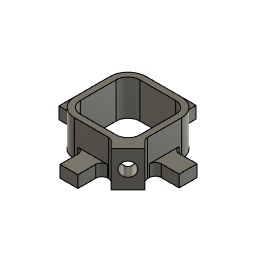
Miniscope_v4_Baseplate_Var_2 (Autodesk Fusion 360 design; units mm, degrees)
Autodesk Fusion 360 part; units mm, degrees
sketch "Sketch1" plane through (0, 0, 0) normal (0, 1, 0) x (1, 0, 0)
  line L0 (1.5, -2) -> (-1.5, -2)
  line L1 (-2, -1.5) -> (-2, 1.5)
  line L2 (-1.5, 2) -> (1.5, 2)
  line L3 (2, 1.5) -> (2, -1.5)
  line L4 (2, -2) -> (-2, 2) construction
  line L5 (-2, -2) -> (2, 2) construction
  line L6 (-1.5, -3) -> (1.5858, -3)
  line L7 (3, -1.5858) -> (3, 1.5)
  line L8 (1.5, 3) -> (-1.5, 3)
  line L9 (-3, 1.5) -> (-3, -1.5)
  line L10 (-3, -3) -> (3, 3) construction
  line L11 (3, -3) -> (-2.9939, 2.9939) construction
  arc A0 (-1.5, 2) -> (-2, 1.5) centre (-1.5, 1.5) ccw
  arc A1 (-2, -1.5) -> (-1.5, -2) centre (-1.5, -1.5) ccw
  arc A2 (1.5, -2) -> (2, -1.5) centre (1.5, -1.5) ccw
  arc A3 (2, 1.5) -> (1.5, 2) centre (1.5, 1.5) ccw
  arc A4 (-1.5, 3) -> (-3, 1.5) centre (-1.5, 1.5) ccw
  arc A5 (-3, -1.5) -> (-1.5, -3) centre (-1.5, -1.5) ccw
  arc A6 (3, 1.5) -> (1.5, 3) centre (1.5, 1.5) ccw
  line L12 (3.7071, -2.2929) -> (2.2929, -3.7071)
  line L13 (2.2929, -3.7071) -> (1.5858, -3)
  line L14 (3, -1.5858) -> (3.7071, -2.2929)
  dimension "d1" = 4
  dimension "d2" = 4
  dimension "d3" = 0.5
  dimension "d4" = 6
  dimension "d5" = 6
  dimension "d6" = 1.5
  dimension "d7" = 2
  dimension "d31" = 2
  dimension "d32" = 3
  constraint perpendicular L0 L1
  constraint parallel L0 L2
  constraint parallel L1 L3
  constraint horizontal L0
  constraint coincident L4 origin
  constraint coincident L5 origin
  constraint perpendicular L6 L7
  constraint parallel L6 L8
  constraint parallel L7 L9
  constraint horizontal L6
  constraint coincident L10 origin
  constraint coincident L11 origin
  constraint coincident L4.end L2
  constraint coincident L4.end L1
  constraint tangent L2 A0
  constraint tangent L1 A0
  constraint coincident L5.start L1
  constraint coincident L5.start L0
  constraint tangent L1 A1
  constraint tangent L0 A1
  constraint equal A0 A1
  constraint tangent L0 A2
  constraint tangent L3 A2
  constraint equal A0 A2
  constraint coincident L5.end L3
  constraint coincident L5.end L2
  constraint tangent L3 A3
  constraint tangent L2 A3
  constraint equal A0 A3
  constraint tangent L8 A4
  constraint tangent L9 A4
  constraint coincident L10.start L9
  constraint coincident L10.start L6
  constraint tangent L9 A5
  constraint tangent L6 A5
  constraint equal A4 A5
  constraint coincident L11.start L6
  constraint coincident L11.start L7
  constraint coincident L10.end L7
  constraint coincident L10.end L8
  constraint tangent L7 A6
  constraint tangent L8 A6
  constraint equal A4 A6
  constraint perpendicular L12 L13
  constraint parallel L13 L14
  constraint midpoint L11.start L12
  constraint parallel L11 L13
  constraint coincident L7.start L14.start
  constraint coincident L6.end L13.end
  measures "d1" distance of L5.start L4.end
  measures "d2" distance of L4.end L5.end
  measures "d3" radius of A0
  measures "d4" distance of L10.start L11.start
  measures "d5" distance of L11.start L10.end
  measures "d6" radius of A4
  measures "d7" distance of L12.start L12.end
  measures "d31" distance of L1 origin
  measures "d32" distance of origin L8
extrude "Extrude1" add sketch "Sketch1" along normal blind 2.5
sketch "Sketch2" plane through (3, 0, 3) normal (0.707107, 0, 0.707107) x (0.707107, 0, -0.707107)
  line L0 (-1, 0) -> (1, 0)
  line L1 (1, 0) -> (1, 2.5)
  line L2 (1, 2.5) -> (-1, 2.5)
  line L3 (-1, 2.5) -> (-1, 0)
  circle A0 centre (0, 1.5) radius 0.595
  dimension "d10" = 1.19
  dimension "d11" = 1.5
  measures "d10" diameter of A0
  measures "d11" distance of L0 A0.centre
extrude "Extrude2" cut sketch "Sketch2" against normal blind 3.4 contours A0
sketch "Sketch4" plane through (0, 0, 0) normal (0, -1, 0) x (1, 0, 0)
  arc A0 (2, 1.5) -> (1.5, 2) centre (1.5, 1.5) ccw
  line L0 (2, 1.5) -> (2, -1.5)
  arc A1 (1.5, -2) -> (2, -1.5) centre (1.5, -1.5) ccw
  line L1 (1.5, -2) -> (-1.5, -2)
  arc A2 (-2, -1.5) -> (-1.5, -2) centre (-1.5, -1.5) ccw
  line L2 (-2, -1.5) -> (-2, 1.5)
  arc A3 (-1.5, 2) -> (-2, 1.5) centre (-1.5, 1.5) ccw
  line L3 (-1.5, 2) -> (1.5, 2)
  line L4 (3, 1.5858) -> (3.7071, 2.2929)
  line L5 (3.7071, 2.2929) -> (2.2929, 3.7071)
  line L6 (2.2929, 3.7071) -> (1.5858, 3)
  line L7 (1.5858, 3) -> (-1.5, 3)
  arc A4 (-1.5, 3) -> (-3, 1.5) centre (-1.5, 1.5) ccw
  line L8 (-3, 1.5) -> (-3, -1.5)
  arc A5 (-3, -1.5) -> (-1.5, -3) centre (-1.5, -1.5) ccw
  line L9 (-1.5, -3) -> (1.5, -3)
  arc A6 (1.5, -3) -> (3, -1.5) centre (1.5, -1.5) ccw
  line L10 (3, -1.5) -> (3, 1.5858)
  line L11 (-0.7071, 5) -> (0.7929, 5)
  line L12 (0.7929, 5) -> (0.7929, 3)
  line L13 (-0.7071, 3) -> (-0.7071, 5)
  line L14 (-0.7071, 5) -> (0.6239, 1.4506) construction
  line L15 (0.7929, 5) -> (-0.5381, 1.4506) construction
  line L16 (-5, -0.7071) -> (-1.4506, 0.6239) construction
  line L17 (-5, -0.7071) -> (-5, 0.7929)
  line L18 (-5, 0.7929) -> (-1.4506, -0.5381) construction
  line L19 (-3, -0.7071) -> (-5, -0.7071)
  line L20 (-5, 0.7929) -> (-3, 0.7929)
  line L21 (0.7071, -5) -> (-0.6239, -1.4506) construction
  line L22 (0.7071, -5) -> (-0.7929, -5)
  line L23 (-0.7929, -5) -> (0.5381, -1.4506) construction
  line L24 (0.7071, -3) -> (0.7071, -5)
  line L25 (-0.7929, -5) -> (-0.7929, -3)
  line L26 (5, 0.7071) -> (1.4506, -0.6239) construction
  line L27 (5, 0.7071) -> (5, -0.7929)
  line L28 (5, -0.7929) -> (1.4506, 0.5381) construction
  line L29 (3, 0.7071) -> (5, 0.7071)
  line L30 (5, -0.7929) -> (3, -0.7929)
  line L31 (0.0429, 3) -> (0.0429, 5) construction
  line L32 (0.6239, 1.4506) -> (-0.5381, 1.4506)
  point P0 (0.0429, 3)
  point P1 (-3, 0.0429)
  point P2 (-0.0429, -3)
  point P3 (3, -0.0429)
  dimension "d26" = 360
  dimension "d29" = 1.5
  dimension "d30" = 2
  constraint perpendicular L11 L12
  constraint parallel L12 L13
  constraint horizontal L11
  constraint coincident L14 P0
  constraint coincident L15 P0
  constraint midpoint L7 P0
  constraint coincident L7 L13.start
  constraint coincident L7 L12.end
  constraint coincident P0 L31.start
  constraint midpoint L11 L31.end
  constraint vertical L31
  constraint horizontal L32
  measures "d29" distance of L11.start L11.end
  measures "d30" distance of L11.end L12.end
extrude "Extrude4" add sketch "Sketch4" against normal blind 1 contours L10 L27 L29 L30 | L7 L11 L12 L13 | L9 L22 L24 L25 | L8 L17 L19 L20
fillet "Fillet2" radius 0.5 8 edges at (3, 0.5, 0.7071) (0.7929, 0.5, 3) (3, 0.5, -0.7929) (0.7071, 0.5, -3) (-0.7929, 0.5, -3) (-3, 0.5, -0.7071) (-0.7071, 0.5, 3) (-3, 0.5, 0.7929)
fillet "Fillet3" radius 0.5 2 edges at (1.5858, 1.25, 3) (3, 1.25, 1.5858)
extrude "Extrude5" add 1 faces at (2.3333, 2.5, 0.4596) along direction (0, 1, 0) blind 0.5
sketch "Sketch6" plane through (0, 3, 0) normal (0, 1, 0) x (-1, 0, 0)
  arc A0 (-1.5, 2) -> (-2, 1.5) centre (-1.5, 1.5) ccw
  line L0 (-1.5, 2) -> (1.5, 2)
  arc A1 (2, 1.5) -> (1.5, 2) centre (1.5, 1.5) ccw
  line L1 (2, 1.5) -> (2, -1.5)
  arc A2 (1.5, -2) -> (2, -1.5) centre (1.5, -1.5) ccw
  line L2 (1.5, -2) -> (-1.5, -2)
  arc A3 (-2, -1.5) -> (-1.5, -2) centre (-1.5, -1.5) ccw
  line L3 (-2, -1.5) -> (-2, 1.5)
  arc A4 (-3, -1.5) -> (-1.5, -3) centre (-1.5, -1.5) ccw
  line L4 (-1.5, -3) -> (1.5, -3)
  arc A5 (1.5, -3) -> (3, -1.5) centre (1.5, -1.5) ccw
  line L5 (3, -1.5) -> (3, 1.5)
  arc A6 (3, 1.5) -> (1.5, 3) centre (1.5, 1.5) ccw
  line L6 (1.5, 3) -> (-1.3787, 3)
  arc A7 (-1.7322, 3.1464) -> (-1.3787, 3) centre (-1.3787, 3.5) ccw
  line L7 (-1.7322, 3.1464) -> (-2.2929, 3.7071)
  line L8 (-2.2929, 3.7071) -> (-3.7071, 2.2929)
  line L9 (-3.7071, 2.2929) -> (-3.1464, 1.7322)
  arc A8 (-3, 1.3787) -> (-3.1464, 1.7322) centre (-3.5, 1.3787) ccw
  line L10 (-3, 1.3787) -> (-3, -1.5)
  line L11 (1.5, 2.5) -> (-1.5, 2.5)
  line L12 (-2.5, 1.5) -> (-2.5, -1.5)
  line L13 (-1.5, -2.5) -> (1.5, -2.5)
  line L14 (2.5, -1.5) -> (2.5, 1.5)
  line L15 (2.5, 2.5) -> (-2.5, -2.5) construction
  line L16 (-2.5, 2.5) -> (2.5, -2.5) construction
  arc A9 (1.5, -2.5) -> (2.5, -1.5) centre (1.5, -1.5) ccw
  arc A10 (2.5, 1.5) -> (1.5, 2.5) centre (1.5, 1.5) ccw
  arc A11 (-1.5, 2.5) -> (-2.5, 1.5) centre (-1.5, 1.5) ccw
  arc A12 (-2.5, -1.5) -> (-1.5, -2.5) centre (-1.5, -1.5) ccw
  dimension "d36" = 0.5
  dimension "d37" = 0.5
  dimension "d38" = 1
  constraint perpendicular L11 L12
  constraint parallel L11 L13
  constraint parallel L12 L14
  constraint horizontal L11
  constraint coincident L15 origin
  constraint coincident L16 origin
  constraint coincident L16.end L13
  constraint coincident L16.end L14
  constraint tangent L13 A9
  constraint tangent L14 A9
  constraint coincident L15.start L14
  constraint coincident L15.start L11
  constraint tangent L14 A10
  constraint tangent L11 A10
  constraint equal A9 A10
  constraint coincident L16.start L11
  constraint coincident L16.start L12
  constraint tangent L11 A11
  constraint tangent L12 A11
  constraint equal A9 A11
  constraint coincident L15.end L12
  constraint coincident L15.end L13
  constraint tangent L12 A12
  constraint tangent L13 A12
  constraint equal A9 A12
  measures "d36" distance of L4 L13
  measures "d37" distance of L5 L14
  measures "d38" radius of A9
extrude "Extrude6" cut sketch "Sketch6" against normal blind 3 contours L11 L12 L13 L14 A9 A10 A11 A12
